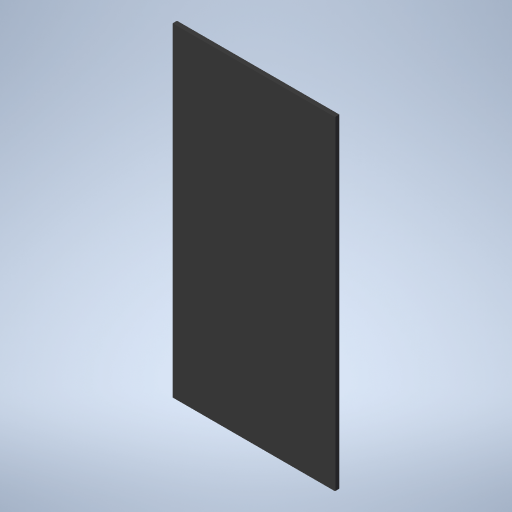
# Autodesk Inventor part: Kicker Poly Top Part
Saved by Autodesk Inventor 2023 (Build 270158000, 158)
## iProperties
Created: 2024-03-11
Part Number: Kicker Poly Top Part
Material: Generic
Document SubType Name: Modeling
Designer: Robodox
Density: 1 g/cm^3
Appearance: Default
Author: Robodox
Autodesk Inventor part; units mm, degrees
ref_plane "YZ Plane" through (0, 0, 0) normal (1, 0, 0) x (0, 1, 0)
ref_plane "XZ Plane" through (0, 0, 0) normal (0, 1, 0) x (-1, 0, 0)
ref_plane "XY Plane" through (0, 0, 0) normal (0, 0, 1) x (1, 0, 0)
sketch "Sketch1" plane through (0, 0, 0) normal (0, 0, 1) x (1, 0, 0)
  line L0 (-39.8758, 37.0237) -> (23.6242, 37.0237)
  line L1 (23.6242, 37.0237) -> (23.6242, -89.9763)
  line L2 (23.6242, -89.9763) -> (-39.8758, -89.9763)
  line L3 (-39.8758, -89.9763) -> (-39.8758, 37.0237)
  point P0 (0, 0)
  dimension "d0" = 63.5
  dimension "d1" = 127
  constraints: 8 end point, 2 parallel, 1 horizontal, 1 perpendicular
  measures "d0" distance of L0.start L0.end
  measures "d1" distance of L2.end L0.start
extrude "Extrusion1" add sketch "Sketch1" along normal blind 1.5875
body "Solid1"
